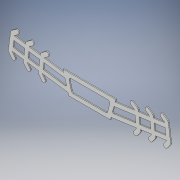
# Autodesk Inventor part: surgical_mask_strap
Saved by Autodesk Inventor 2019 (Build 230136000, 136)
## iProperties
Created: 2020-03-28
Part Number: surgical_mask_strap
Material: Generic
Document SubType Name: Modeling
Designer: tdeith
Density: 1 g/cm^3
Appearance: Default
Author: tdeith
Autodesk Inventor part; units mm, degrees
ref_plane "YZ Plane" through (0, 0, 0) normal (1, 0, 0) x (0, 1, 0)
ref_plane "XZ Plane" through (0, 0, 0) normal (0, 1, 0) x (-1, 0, 0)
ref_plane "XY Plane" through (0, 0, 0) normal (0, 0, 1) x (1, 0, 0)
sketch "Sketch2" plane through (0, 0, 0) normal (0, 0, 1) x (1, 0, 0)
  line L0 (77.9266, 27.07) -> (80.5163, 8.6427)
  line L1 (79.2214, 17.8564) -> (4.7951, 7.3964) construction
  line L2 (26, 20) -> (-26, 20)
  line L3 (-20.641, 0) -> (20.641, 0)
  line L4 (-48.887, 0) -> (111.3221, 0) construction
  line L5 (0, 23.1256) -> (0, -5.1147) construction
  line L6 (0, -5.1147) -> (0, -6.596)
  line L7 (-20.641, 0) -> (-26, 20)
  line L8 (26, 20) -> (20.641, 0)
  line L9 (25.3301, 17.5) -> (78.2267, 24.9341)
  line L10 (80.2162, 10.7786) -> (21.3109, 2.5)
  line L11 (0, -14.2946) -> (0, 39.5956) projected
  line L12 (24.2054, 13.3026) -> (78.7834, 20.9731)
  line L13 (79.6595, 14.7397) -> (22.4356, 6.6974)
  line L14 (69.1136, 28.7025) -> (74.1961, 24.8726)
  line L15 (76.3247, 9.7268) -> (72.4947, 4.6443)
  line L16 (72.4947, 4.6443) -> (75.6893, 2.237)
  line L17 (75.6893, 2.237) -> (80.5163, 8.6427)
  line L18 (77.9266, 27.07) -> (71.5208, 31.897)
  line L19 (71.5208, 31.897) -> (69.1136, 28.7025)
  line L20 (74.1961, 24.8726) -> (74.2657, 24.3774)
  line L21 (74.8224, 20.4164) -> (75.6984, 14.183)
  line L22 (76.2551, 10.2219) -> (76.3247, 9.7268)
  line L23 (77.9266, 27.07) -> (74.1961, 24.8726) construction
  point P0 (0, 6.7225)
  point P1 (88.4351, 19.1513)
  dimension "d28" = 82
  dimension "d30" = 80
  dimension "d37" = 4
  dimension "d39" = 4
  dimension "d40" = 5
  dimension "d58" = 2.5
  dimension "d59" = 26
  dimension "d60" = 105
  dimension "d63" = 2.5
  dimension "d64" = 20
  dimension "d67" = 4
  dimension "d68" = 0.5
  constraints: 44 end point, 20 point on line, 9 parallel, 4 collinear, 3 perpendicular, 2 symmetric about line, 1 midpoint, 1 vertical, 4 other
  measures "d28" angle of L5 L1
  measures "d30" distance from line of point (0, 6.723) L0
  measures "d37" distance between parallel lines of L9 L12
  measures "d39" distance between parallel lines of L14 L18
  measures "d40" distance from line of L9 L14.start
  measures "d58" distance from line of L2 L9.start
  measures "d59" distance from line of L2.end L11
  measures "d60" angle of L4 L7
  measures "d63" distance from line of L4 L10.end
  measures "d64" distance between parallel lines of L3 L2
  measures "d67" distance between parallel lines of L0 L21
  measures "d68" distance from line of L9 L14.end
extrude "Extrusion2" add sketch "Sketch2" along normal blind 1 contours L8 L3 L11 L2 | L11 L3 L7 L2
sketch "Sketch3" plane through (0, 0, 1) normal (0, 0, 1) x (1, 0, 0)
  line L0 (26, 20) -> (-26, 20) projected
  line L1 (-26, 20) -> (-20.641, 0) projected
  line L2 (-20.641, 0) -> (20.641, 0) projected
  line L3 (20.641, 0) -> (26, 20) projected
  line L4 (-18.1806, 16) -> (18.1806, 16)
  line L5 (20.1125, 13.4824) -> (17.9689, 5.4824)
  line L6 (16.0371, 4) -> (-16.0371, 4)
  line L7 (-17.9689, 5.4824) -> (-20.1125, 13.4824)
  arc A0 (-18.1806, 16) -> (-20.1125, 13.4824) centre (-18.1806, 14) ccw
  arc A1 (-17.9689, 5.4824) -> (-16.0371, 4) centre (-16.0371, 6) ccw
  arc A2 (16.0371, 4) -> (17.9689, 5.4824) centre (16.0371, 6) ccw
  arc A3 (20.1125, 13.4824) -> (18.1806, 16) centre (18.1806, 14) ccw
  point P0 (0, 0)
  dimension "d33" = 4
  dimension "d34" = 2
  constraints: 8 end point, 8 point on circle, 8 tangent, 4 centre point, 3 equal radius, 3 other
  measures "d33" distance between parallel lines of L0 L4
  measures "d34" radius of A0
extrude "Extrusion3" cut sketch "Sketch3" against normal through all contours L4 A3 L5 A2 L6 A1 L7 A0
extrude "Extrusion4" add sketch "Sketch2" along normal blind 1 contours L0 L12 L8 L9 | L0 L10 L8 L13
extrude "Extrusion6" add sketch "Sketch2" along normal blind 1 contours L0 L9 L20 L14 L19 L18 | L0 L13 L21 L12 | L0 L17 L16 L15 L22 L10
fillet "Fillet2" radius 2 6 edges at (72.4947, 4.6443, 0.5) (75.6893, 2.237, 0.5) (80.5163, 8.6427, 0.5) (69.1136, 28.7025, 0.5) (71.5208, 31.897, 0.5) (77.9266, 27.07, 0.5)
fillet "Fillet4" radius 1 3 edges at (24.2054, 13.3026, 0.5) (22.4356, 6.6974, 0.5) (21.3109, 2.5, 0.5)
pattern_linear "Rectangular Pattern1" count 3 spacing 15 along (-0.9902681, -0.1391731, 0) of "Fillet2", "Extrusion6"
mirror "Mirror2" about plane through (0, 0, 0) normal (1, 0, 0)
body "Solid1"
body "Solid2"
